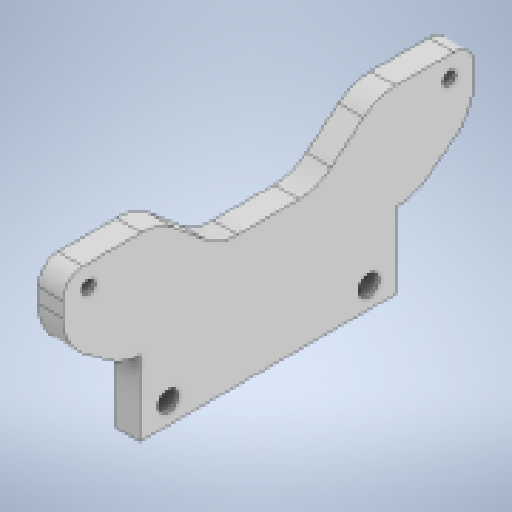
# Autodesk Inventor part: Camera_mount
Saved by Autodesk Inventor 2024.2 (Build 282272000, 272)
## iProperties
Created: 2024-01-14
Part Number: Camera_mount
Material: Generic
Document SubType Name: Modeling
Designer: 박동준
Density: 1 g/cm^3
Appearance: Default
Author: 박동준
Autodesk Inventor part; units mm, degrees
ref_plane "YZ Plane" through (0, 0, 0) normal (1, 0, 0) x (0, 1, 0)
ref_plane "XZ Plane" through (0, 0, 0) normal (0, 1, 0) x (-1, 0, 0)
ref_plane "XY Plane" through (0, 0, 0) normal (0, 0, 1) x (1, 0, 0)
sketch "Sketch1" plane through (0, 0, 0) normal (1, 0, 0) x (0, 1, 0)
  line L0 (41, 41) -> (-41, 41)
  line L1 (-41, 41) -> (-41, -41)
  line L2 (-41, -41) -> (41, -41)
  line L3 (41, -41) -> (41, 41)
  point P0 (0, 0)
  point P1 (0, 41)
  point P2 (41, 0)
  dimension "d0" = 82
  dimension "d1" = 82
  constraints: 8 end point, 2 midpoint, 2 parallel, 1 horizontal, 1 horizontal alignment, 1 perpendicular, 1 vertical alignment
  measures "d0" distance of L0.end L1.end
  measures "d1" distance of L0.start L0.end
extrude "Extrusion1" add sketch "Sketch1" along normal mid plane 2
sketch "Sketch2" plane through (-1, 0, 0) normal (-1, 0, 0) x (0, 0, 1)
  line L0 (31.6667, 22) -> (37, 26) projected
  arc A0 (25.6667, 20) -> (31.6667, 22) centre (25.6667, 30) ccw projected
  line L1 (17.5, 20) -> (25.6667, 20) projected
  line L2 (17.5, 20) -> (17.5, 18.2355) projected
  line L3 (-17.5, 18.2356) -> (17.5, 18.2356) projected
  line L4 (-17.5, 20) -> (-17.5, 18.2355) projected
  line L5 (-25.6667, 20) -> (-17.5, 20) projected
  arc A1 (-31.6667, 22) -> (-25.6667, 20) centre (-25.6667, 30) ccw projected
  line L6 (-37, 26) -> (-31.6667, 22) projected
  arc A2 (-41, 34) -> (-37, 26) centre (-31, 34) ccw projected
  line L7 (-41, 37) -> (-41, 34) projected
  arc A3 (-37, 41) -> (-41, 37) centre (-37, 37) ccw projected
  line L8 (-37, 41) -> (-25.3705, 41) projected
  arc A4 (-18.9687, 38.6822) -> (-25.3705, 41) centre (-25.3705, 31) ccw projected
  line L9 (-18.9687, 38.6822) -> (-12.5313, 33.3178) projected
  arc A5 (-12.5313, 33.3178) -> (-6.1295, 31) centre (-6.1295, 41) ccw projected
  line L10 (-6.1295, 31) -> (6.1295, 31) projected
  arc A6 (6.1295, 31) -> (12.5313, 33.3178) centre (6.1295, 41) ccw projected
  line L11 (12.5313, 33.3178) -> (18.9687, 38.6822) projected
  arc A7 (25.3705, 41) -> (18.9687, 38.6822) centre (25.3705, 31) ccw projected
  line L12 (25.3705, 41) -> (37, 41) projected
  arc A8 (41, 37) -> (37, 41) centre (37, 37) ccw projected
  line L13 (41, 37) -> (41, 34) projected
  arc A9 (37, 26) -> (41, 34) centre (31, 34) ccw projected
  circle A10 centre (36, 36.9) radius 1.35 projected
  circle A11 centre (-36, 36.9) radius 1.35 projected
  line L14 (-25.6667, 20) -> (-25.6667, 5)
  line L15 (25.6667, 20) -> (25.6667, 5)
  line L16 (25.6667, 5) -> (-25.6667, 5)
  point P0 (0, 0)
  dimension "d4" = 15
  constraints: 6 end point, 2 vertical, 1 perpendicular
  measures "d4" distance of L5.start L14.end
extrude "Extrusion2" add sketch "Sketch2" along normal blind 2
sketch "Sketch3" plane through (1, 0, 0) normal (1, 0, 0) x (0, 0, -1)
  line L0 (-31.6667, 22) -> (-37, 26) projected
  arc A0 (-41, 34) -> (-37, 26) centre (-31, 34) ccw projected
  line L1 (-41, 34) -> (-41, 37) projected
  arc A1 (-37, 41) -> (-41, 37) centre (-37, 37) ccw projected
  line L2 (-37, 41) -> (-25.3705, 41) projected
  arc A2 (-18.9687, 38.6822) -> (-25.3705, 41) centre (-25.3705, 31) ccw projected
  line L3 (-18.9687, 38.6822) -> (-12.5313, 33.3178) projected
  arc A3 (-12.5313, 33.3178) -> (-6.1295, 31) centre (-6.1295, 41) ccw projected
  line L4 (-6.1295, 31) -> (6.1295, 31) projected
  arc A4 (6.1295, 31) -> (12.5313, 33.3178) centre (6.1295, 41) ccw projected
  line L5 (12.5313, 33.3178) -> (18.9687, 38.6822) projected
  arc A5 (25.3705, 41) -> (18.9687, 38.6822) centre (25.3705, 31) ccw projected
  line L6 (25.3705, 41) -> (37, 41) projected
  arc A6 (41, 37) -> (37, 41) centre (37, 37) ccw projected
  line L7 (41, 37) -> (41, 34) projected
  arc A7 (37, 26) -> (41, 34) centre (31, 34) ccw projected
  line L8 (37, 26) -> (31.6667, 22) projected
  arc A8 (25.6667, 20) -> (31.6667, 22) centre (25.6667, 30) ccw projected
  line L9 (25.6667, 20) -> (25.6667, 5) projected
  line L10 (25.6667, 5) -> (-25.6667, 5) projected
  line L11 (-25.6667, 5) -> (-25.6667, 20) projected
  arc A9 (-31.6667, 22) -> (-25.6667, 20) centre (-25.6667, 30) ccw projected
  circle A10 centre (-36, 36.9) radius 1.35 projected
  circle A11 centre (36, 36.9) radius 1.35 projected
  line L12 (-41, -41) -> (41, -41) projected
  line L13 (41, -41) -> (41, 41) projected
  line L14 (41, 41) -> (-41, 41) projected
  line L15 (-41, 41) -> (-41, -41) projected
  point P0 (0, 0)
  point P1 (41, 37)
  point P2 (-37, 41)
  point P3 (25.3705, 41)
  point P4 (-41, 34)
extrude "Extrusion3" cut sketch "Sketch3" against normal blind 15 contours A9 L11 L10 L9 A8 L8 A7 L13 L12 L15 A0 L0 | L15 L14 A1 | L14 A5 L5 A4 L4 A3 L3 A2 | A6 L14 L13
sketch "Sketch4" plane through (-3, 0, 0) normal (-1, 0, 0) x (0, 0, 1)
  line L0 (31.6667, 22) -> (37, 26) projected
  arc A0 (37, 26) -> (41, 34) centre (31, 34) ccw projected
  line L1 (41, 34) -> (41, 37) projected
  arc A1 (41, 37) -> (37, 41) centre (37, 37) ccw projected
  line L2 (37, 41) -> (25.3705, 41) projected
  arc A2 (25.3705, 41) -> (18.9687, 38.6822) centre (25.3705, 31) ccw projected
  line L3 (18.9687, 38.6822) -> (12.5313, 33.3178) projected
  arc A3 (6.1295, 31) -> (12.5313, 33.3178) centre (6.1295, 41) ccw projected
  line L4 (6.1295, 31) -> (-6.1295, 31) projected
  arc A4 (-12.5313, 33.3178) -> (-6.1295, 31) centre (-6.1295, 41) ccw projected
  line L5 (-12.5313, 33.3178) -> (-18.9687, 38.6822) projected
  arc A5 (-18.9687, 38.6822) -> (-25.3705, 41) centre (-25.3705, 31) ccw projected
  line L6 (-25.3705, 41) -> (-37, 41) projected
  arc A6 (-37, 41) -> (-41, 37) centre (-37, 37) ccw projected
  line L7 (-41, 37) -> (-41, 34) projected
  arc A7 (-41, 34) -> (-37, 26) centre (-31, 34) ccw projected
  line L8 (-37, 26) -> (-31.6667, 22) projected
  arc A8 (-31.6667, 22) -> (-25.6667, 20) centre (-25.6667, 30) ccw projected
  line L9 (-25.6667, 20) -> (-25.6667, 5) projected
  line L10 (-25.6667, 5) -> (25.6667, 5) projected
  line L11 (25.6667, 5) -> (25.6667, 20) projected
  arc A9 (25.6667, 20) -> (31.6667, 22) centre (25.6667, 30) ccw projected
  circle A10 centre (36, 36.9) radius 1.35 projected
  circle A11 centre (-36, 36.9) radius 1.35 projected
  circle A12 centre (-36, 36.9) radius 2.3
  circle A13 centre (36, 36.9) radius 2.3
  point P0 (0, 0)
  dimension "d9" = 4.6
  dimension "d10" = 4.6
  constraints: 2 centre point, 2 coincident
  measures "d9" diameter of A12
  measures "d10" diameter of A13
extrude "Extrusion4" cut sketch "Sketch4" against normal blind 1.4 contours A12 | A13
sketch "Sketch5" plane through (-3, 0, 0) normal (-1, 0, 0) x (0, 0, 1)
  circle A0 centre (36, 36.9) radius 2.3 projected
  circle A1 centre (-36, 36.9) radius 2.3 projected
  line L0 (31.6667, 22) -> (37, 26) projected
  arc A2 (37, 26) -> (41, 34) centre (31, 34) ccw projected
  line L1 (41, 34) -> (41, 37) projected
  arc A3 (41, 37) -> (37, 41) centre (37, 37) ccw projected
  line L2 (37, 41) -> (25.3705, 41) projected
  arc A4 (25.3705, 41) -> (18.9687, 38.6822) centre (25.3705, 31) ccw projected
  line L3 (18.9687, 38.6822) -> (12.5313, 33.3178) projected
  arc A5 (6.1295, 31) -> (12.5313, 33.3178) centre (6.1295, 41) ccw projected
  line L4 (6.1295, 31) -> (-6.1295, 31) projected
  arc A6 (-12.5313, 33.3178) -> (-6.1295, 31) centre (-6.1295, 41) ccw projected
  line L5 (-12.5313, 33.3178) -> (-18.9687, 38.6822) projected
  arc A7 (-18.9687, 38.6822) -> (-25.3705, 41) centre (-25.3705, 31) ccw projected
  line L6 (-25.3705, 41) -> (-37, 41) projected
  arc A8 (-37, 41) -> (-41, 37) centre (-37, 37) ccw projected
  line L7 (-41, 37) -> (-41, 34) projected
  arc A9 (-41, 34) -> (-37, 26) centre (-31, 34) ccw projected
  line L8 (-37, 26) -> (-31.6667, 22) projected
  arc A10 (-31.6667, 22) -> (-25.6667, 20) centre (-25.6667, 30) ccw projected
  line L9 (-25.6667, 20) -> (-25.6667, 5) projected
  line L10 (-25.6667, 5) -> (25.6667, 5) projected
  line L11 (25.6667, 5) -> (25.6667, 20) projected
  arc A11 (25.6667, 20) -> (31.6667, 22) centre (25.6667, 30) ccw projected
  circle A12 centre (-36, 36.9) radius 1.3
  circle A13 centre (36, 36.9) radius 1.3
  point P0 (0, 0)
  dimension "d13" = 2.6
  dimension "d14" = 2.6
  constraints: 2 centre point, 2 coincident
  measures "d13" diameter of A12
  measures "d14" diameter of A13
extrude "Extrusion5" cut sketch "Sketch5" against normal through all contours A12 | A13
sketch "Sketch6" plane through (1, 0, 0) normal (1, 0, 0) x (0, 0, -1)
  arc A0 (-37, 41) -> (-41, 37) centre (-37, 37) ccw projected
  line L0 (-41, 37) -> (-41, 34) projected
  arc A1 (-41, 34) -> (-37, 26) centre (-31, 34) ccw projected
  line L1 (-37, 26) -> (-31.6667, 22) projected
  arc A2 (-31.6667, 22) -> (-25.6667, 20) centre (-25.6667, 30) ccw projected
  line L2 (-25.6667, 20) -> (-25.6667, 5) projected
  line L3 (-25.6667, 5) -> (25.6667, 5) projected
  line L4 (25.6667, 5) -> (25.6667, 20) projected
  arc A3 (25.6667, 20) -> (31.6667, 22) centre (25.6667, 30) ccw projected
  line L5 (31.6667, 22) -> (37, 26) projected
  arc A4 (37, 26) -> (41, 34) centre (31, 34) ccw projected
  line L6 (41, 34) -> (41, 37) projected
  arc A5 (41, 37) -> (37, 41) centre (37, 37) ccw projected
  line L7 (37, 41) -> (25.3705, 41) projected
  arc A6 (25.3705, 41) -> (18.9687, 38.6822) centre (25.3705, 31) ccw projected
  line L8 (18.9687, 38.6822) -> (12.5313, 33.3178) projected
  arc A7 (6.1295, 31) -> (12.5313, 33.3178) centre (6.1295, 41) ccw projected
  line L9 (6.1295, 31) -> (-6.1295, 31) projected
  arc A8 (-12.5313, 33.3178) -> (-6.1295, 31) centre (-6.1295, 41) ccw projected
  line L10 (-12.5313, 33.3178) -> (-18.9687, 38.6822) projected
  arc A9 (-18.9687, 38.6822) -> (-25.3705, 41) centre (-25.3705, 31) ccw projected
  line L11 (-25.3705, 41) -> (-37, 41) projected
  circle A10 centre (-20, 9.2) radius 2.05
  circle A11 centre (20, 9.2) radius 2.05
  line L12 (-20, 9.2) -> (20, 9.2) construction
  point P0 (0, 0)
  point P1 (0, 31)
  point P2 (0, 9.2)
  dimension "d17" = 4.1
  dimension "d18" = 4.1
  dimension "d19" = 4.2
  dimension "d20" = 40
  constraints: 2 centre point, 2 end point, 2 midpoint, 1 horizontal, 1 vertical alignment
  measures "d17" diameter of A10
  measures "d18" diameter of A11
  measures "d19" distance between parallel lines of L3 L12
  measures "d20" distance of L12.end L12.start
extrude "Extrusion6" cut sketch "Sketch6" against normal blind 10 contours A10 | A11
fillet "Fillet1" radius 2 4 edges at (-1, 20, -25.6667) (-1, 5, -25.6667) (-1, 5, 25.6667) (-1, 20, 25.6667)
body "Solid1"
